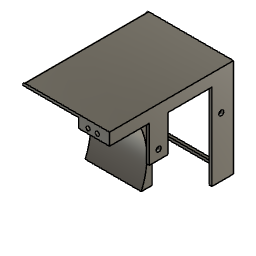
왼쪽 중앙 범퍼 (Autodesk Fusion 360 design; units mm, degrees)
Autodesk Fusion 360 part; units mm, degrees
sketch "스케치1" plane through (0, 0, 0) normal (0, 1, 0) x (1, 0, 0)
  line L0 (-46.5, -52.5) -> (46.5, -52.5)
  line L1 (46.5, -52.5) -> (46.5, 52.5)
  line L2 (46.5, 52.5) -> (-46.5, 52.5)
  line L3 (-46.5, 52.5) -> (-46.5, -52.5)
  line L4 (-46.5, -52.5) -> (46.5, 52.5) construction
  line L5 (46.5, -52.5) -> (-46.5, 52.5) construction
  line L6 (0, -52.5) -> (0, -47.5)
  line L7 (0, 52.5) -> (0, 49.5)
  line L8 (46.5, 0) -> (38.5, 0)
  line L9 (-46.5, 0) -> (-40.5, 0)
  line L10 (-40.5, 0) -> (-40.5, -47.5)
  line L11 (-40.5, -47.5) -> (38.5, -47.5)
  line L12 (38.5, -47.5) -> (38.5, 49.5)
  line L13 (38.5, 49.5) -> (-40.5, 49.5)
  line L14 (-40.5, 49.5) -> (-40.5, 0)
  dimension "d1" = 105
  dimension "d2" = 93
  dimension "d3" = 5
  dimension "d4" = 3
  dimension "d5" = 8
  dimension "d6" = 6
  constraint horizontal L0
  constraint perpendicular L0 L1
  constraint parallel L0 L2
  constraint parallel L1 L3
  constraint coincident L4 origin
  constraint coincident L5 origin
  constraint midpoint L0 L6.start
  constraint perpendicular L0 L6
  constraint midpoint L2 L7.start
  constraint perpendicular L2 L7
  constraint midpoint L1 L8.start
  constraint perpendicular L1 L8
  constraint midpoint L3 L9.start
  constraint perpendicular L3 L9
  constraint perpendicular L9 L10
  constraint perpendicular L6 L11
  constraint perpendicular L2 L12
  constraint perpendicular L12 L13
  constraint perpendicular L9 L14
  measures "d1" distance of L0.end L1.end
  measures "d2" distance of L1.end L2.end
  measures "d3" distance of L6.start L6.end
  measures "d4" distance of L7.start L7.end
  measures "d5" distance of L8.start L8.end
  measures "d6" distance of L9.start L9.end
extrude "돌출1" add sketch "스케치1" along normal blind 132.5 contours L0 L3 L6 L9 L10 L11 | L0 L1 L6 L8 L11 L12 | L2 L3 L7 L9 L13 L14 | L1 L2 L7 L8 L12 L13
sketch "스케치2" plane through (0, 0, 0) normal (0, -1, 0) x (1, 0, 0)
  line L0 (-40.5, -49.5) -> (-40.5, 47.5)
  line L1 (-40.5, 47.5) -> (38.5, 47.5)
  line L2 (38.5, 47.5) -> (38.5, -49.5)
  line L3 (38.5, -49.5) -> (-40.5, -49.5)
  line L4 (-46.5, 52.5) -> (-46.5, -52.5)
  line L5 (-46.5, -52.5) -> (46.5, -52.5)
  line L6 (46.5, -52.5) -> (46.5, 52.5)
  line L7 (46.5, 52.5) -> (-46.5, 52.5)
  line L8 (-46.5, 52.5) -> (-43.5, 52.5)
  line L9 (-43.5, 52.5) -> (-43.5, 49.5)
  line L10 (-43.5, 49.5) -> (-46.5, 49.5)
  line L11 (-46.5, 49.5) -> (-46.5, 52.5)
  line L12 (46.5, -52.5) -> (43.5, -52.5)
  line L13 (-43.5, 49.5) -> (43.5, 49.5)
  line L14 (43.5, 49.5) -> (43.5, -52.5)
  line L15 (43.5, -52.5) -> (-43.5, -52.5)
  line L16 (-43.5, -52.5) -> (-43.5, 49.5)
  dimension "d9" = 3
  dimension "d10" = 3
  dimension "d11" = 3
  constraint horizontal L8
  constraint vertical L9
  constraint horizontal L10
  constraint vertical L11
  constraint coincident L4.start L7.end
  constraint coincident L5.end L6.start
  constraint perpendicular L6 L12
  constraint horizontal L13
  constraint vertical L14
  constraint horizontal L15
  constraint vertical L16
  measures "d9" distance of L4.start L8.end
  measures "d10" distance of L4.start L10.end
  measures "d11" distance of L5.end L12.end
extrude "돌출2" cut sketch "스케치2" against normal blind 129.5 contours L5 L13 L14 L15 L16
sketch "스케치3" plane through (-46.5, 0, 0) normal (-1, 0, 0) x (0, -1, 0)
  line L0 (0, -52.5) -> (0, 52.5)
  line L1 (0, 52.5) -> (-132.5, 52.5)
  line L2 (-132.5, 52.5) -> (-132.5, -52.5)
  line L3 (-132.5, -52.5) -> (0, -52.5)
  line L4 (0, 52.5) -> (0, -23.5)
  circle A0 centre (0, -23.5) radius 73
  circle A1 centre (0, -23.5) radius 75.5
  line L5 (0, 52.5) -> (-42.5, 52.5)
  line L6 (-42.5, 52.5) -> (-42.5, 35.8528)
  line L7 (-42.5, 35.8528) -> (0, 35.8528)
  line L8 (0, 35.8528) -> (0, 52.5)
  line L9 (0, 52.5) -> (-3, 52.5)
  line L10 (-3, 52.5) -> (-3, 49.4383)
  line L11 (-3, 49.4383) -> (0, 49.4383)
  line L12 (0, 49.4383) -> (0, 52.5)
  line L13 (-66.9925, -52.5) -> (-62.9352, -52.5)
  line L14 (-62.9352, -52.5) -> (-62.9352, -49.5)
  line L15 (-62.9352, -49.5) -> (-66.9925, -49.5)
  line L16 (-66.9925, -49.5) -> (-66.9925, -52.5)
  line L17 (0, 52.5) -> (-75.5, 52.5)
  line L18 (-75.5, 52.5) -> (-75.5, -52.5)
  line L19 (-75.5, -52.5) -> (0, -52.5)
  line L20 (0, -52.5) -> (0, 52.5)
  dimension "d14" = 76
  dimension "d15" = 146
  dimension "d16" = 151
  dimension "d45" = 42.5
  dimension "d46" = 3
  dimension "d50" = 3
  dimension "d71" = 75.5
  constraint coincident L0.end L1.start
  constraint perpendicular L1 L4
  constraint coincident L4.end A0.centre
  constraint concentric A0 A1
  constraint horizontal L5
  constraint vertical L6
  constraint horizontal L7
  constraint vertical L8
  constraint coincident A0 L6.end
  constraint horizontal L9
  constraint vertical L10
  constraint horizontal L11
  constraint vertical L12
  constraint coincident A0 L10.end
  constraint horizontal L13
  constraint vertical L14
  constraint horizontal L15
  constraint vertical L16
  constraint coincident A0 L13.start
  constraint coincident L3 L13.start
  constraint horizontal L17
  constraint vertical L18
  constraint horizontal L19
  constraint vertical L20
  measures "d14" distance of L0.end L4.end
  measures "d15" diameter of A0
  measures "d16" diameter of A1
  measures "d45" distance of L0.end L5.end
  measures "d46" distance of L0.end L9.end
  measures "d50" distance of L13.start L15.end
  measures "d71" distance of L0.end L17.end
extrude "돌출3" cut sketch "스케치3" against normal blind 10 contours L0 L3 L4 A0 L7 L14 L15 L16 L19 L20 | L3 L13 L14 L15 L16 L19 | L0 L4 A0 L7 L8 L11 L20 | L0 L4 A0 L8 L11 L12 L20
sketch "스케치4" plane through (0, 132.5, 0) normal (0, 1, 0) x (-1, 0, 0)
  line L0 (40.5, 47.5) -> (40.5, -49.5)
  line L1 (40.5, -49.5) -> (-38.5, -49.5)
  line L2 (-38.5, -49.5) -> (-38.5, 47.5)
  line L3 (-38.5, 47.5) -> (40.5, 47.5)
  line L4 (46.5, -52.5) -> (46.5, 52.5)
  line L5 (46.5, 52.5) -> (-46.5, 52.5)
  line L6 (-46.5, 52.5) -> (-46.5, -52.5)
  line L7 (-46.5, -52.5) -> (46.5, -52.5)
  line L8 (-38.5, -49.5) -> (-38.5, -6.5)
  line L9 (-38.5, -6.5) -> (-28.5, -6.5)
  line L10 (-28.5, -6.5) -> (-28.5, 3.5)
  line L11 (-28.5, 3.5) -> (-38.5, 3.5)
  line L12 (-38.5, 3.5) -> (-38.5, -6.5)
  line L13 (40.5, -6.5) -> (30.5, -6.5)
  line L14 (30.5, -6.5) -> (30.5, 3.5)
  line L15 (30.5, 3.5) -> (40.5, 3.5)
  line L16 (40.5, 3.5) -> (40.5, -6.5)
  circle A0 centre (-33.5, -1.5) radius 2.15
  circle A1 centre (35.5, -1.5) radius 2.15
  dimension "d19" = 43
  dimension "d20" = 10
  dimension "d21" = 10
  dimension "d22" = 10
  dimension "d23" = 10
  dimension "d24" = 4.3
  dimension "d25" = 4.3
  constraint coincident L1.end L2.start
  constraint perpendicular L1 L8
  constraint horizontal L9
  constraint vertical L10
  constraint horizontal L11
  constraint vertical L12
  constraint horizontal L13
  constraint vertical L14
  constraint horizontal L15
  constraint vertical L16
  constraint coincident L0 L13.start
  measures "d19" distance of L1.end L8.end
  measures "d20" distance of L8.end L9.end
  measures "d21" distance of L8.end L11.end
  measures "d22" distance of L13.start L13.end
  measures "d23" distance of L13.start L15.end
  measures "d24" diameter of A0
  measures "d25" diameter of A1
extrude "돌출4" add sketch "스케치4" against normal blind 3 contours L0 L13 L14 L15 L16 | L2 L9 L10 L11 L12
sketch "스케치5" plane through (43.5, 0, 0) normal (-1, 0, 0) x (0, -1, 0)
  line L0 (0, -52.5) -> (0, 49.5)
  line L1 (0, 49.5) -> (-129.5, 49.5)
  line L2 (-129.5, 49.5) -> (-129.5, -52.5)
  line L3 (-129.5, -52.5) -> (0, -52.5)
  line L4 (-129.5, 49.5) -> (-109.5, 49.5)
  line L5 (-109.5, 49.5) -> (-109.5, -52.5)
  line L6 (-109.5, -52.5) -> (-129.5, -52.5)
  line L7 (-129.5, -52.5) -> (-129.5, 49.5)
  line L8 (-109.5, 49.5) -> (-62.5, 49.5)
  line L9 (-62.5, 49.5) -> (-42.5, 49.5)
  line L10 (-42.5, 49.5) -> (-42.5, -52.5)
  line L11 (-42.5, -52.5) -> (-62.5, -52.5)
  line L12 (-62.5, -52.5) -> (-62.5, 49.5)
  line L13 (-42.5, 49.5) -> (-42.5, 20.5)
  line L14 (-109.5, 20.5) -> (-129.5, 20.5)
  line L15 (-129.5, 20.5) -> (-129.5, 0.5)
  line L16 (-129.5, 0.5) -> (-109.5, 0.5)
  line L17 (-109.5, 0.5) -> (-109.5, 20.5)
  circle A0 centre (-119.5, 10.5) radius 2.65
  line L18 (-42.5, 20.5) -> (-62.5, 20.5)
  line L19 (-62.5, 20.5) -> (-62.5, 0.5)
  line L20 (-62.5, 0.5) -> (-42.5, 0.5)
  line L21 (-42.5, 0.5) -> (-42.5, 20.5)
  circle A1 centre (-52.5, 10.5) radius 2.65
  dimension "d28" = 20
  dimension "d29" = 47
  dimension "d30" = 20
  dimension "d31" = 29
  dimension "d33" = 20
  dimension "d34" = 20
  dimension "d36" = 5.3
  dimension "d41" = 20
  dimension "d42" = 5.3
  constraint horizontal L4
  constraint vertical L5
  constraint horizontal L6
  constraint vertical L7
  constraint coincident L1.end L2.start
  constraint perpendicular L5 L8
  constraint horizontal L9
  constraint vertical L10
  constraint horizontal L11
  constraint vertical L12
  constraint perpendicular L1 L13
  constraint horizontal L14
  constraint vertical L15
  constraint horizontal L16
  constraint vertical L17
  constraint coincident L5 L14.start
  constraint horizontal L18
  constraint vertical L19
  constraint horizontal L20
  constraint vertical L21
  measures "d28" distance of L1.end L4.end
  measures "d29" distance of L4.end L8.end
  measures "d30" distance of L8.end L9.end
  measures "d31" distance of L9.end L13.end
  measures "d33" distance of L14.start L14.end
  measures "d34" distance of L14.start L16.end
  measures "d36" diameter of A0
  measures "d41" distance of L13.end L20.end
  measures "d42" diameter of A1
extrude "돌출5" cut sketch "스케치5" against normal blind 3 contours L0 L1 L3 L10 L13 L21 | L3 L10 L11 L12 L20 | L1 L3 L5 L8 L12 L17 L19 | A0 | A1
extrude "돌출19" add sketch "스케치3" against normal blind 60 contours L3 A0 A1 L6 L19 | A0 A1 L6 L10 | L3 A1 L18 L19 | L0 L4 A0 A1 L8 L10 L12 L20 | L1 A1 L5 L6 L10 L17 | L1 A1 L6 L17 L18 | L0 L1 L4 A1 L5 L8 L9 L10 L12 L17 L20
extrude "돌출21" add 1 faces at (-24.5, 75.5, 15.5) along direction (0, 1, 0) blind 3
sketch "스케치12" plane through (0, 0, 49.5) normal (0, 0, -1) x (1, 0, 0)
  line L0 (13.5, -78.5) -> (-43.5, -78.5)
  line L1 (-43.5, -78.5) -> (-43.5, -129.5)
  line L2 (-43.5, -129.5) -> (43.5, -129.5)
  line L3 (43.5, -129.5) -> (43.5, -109.5)
  line L4 (43.5, -109.5) -> (46.5, -109.5)
  line L5 (46.5, -109.5) -> (46.5, -62.5)
  line L6 (46.5, -62.5) -> (43.5, -62.5)
  line L7 (43.5, -62.5) -> (43.5, -42.5)
  line L8 (43.5, -42.5) -> (46.5, -42.5)
  line L9 (46.5, -42.5) -> (46.5, 0)
  line L10 (46.5, 0) -> (13.5, 0)
  line L11 (13.5, 0) -> (13.5, -78.5)
  line L12 (46.5, 0) -> (13.5, 0)
  line L13 (13.5, 0) -> (13.5, -3)
  line L14 (13.5, -3) -> (46.5, -3)
  line L15 (46.5, -3) -> (46.5, 0)
  line L16 (43.5, -129.5) -> (46.5, -129.5)
  line L17 (46.5, -129.5) -> (46.5, 0)
  line L18 (46.5, 0) -> (43.5, 0)
  line L19 (43.5, 0) -> (43.5, -129.5)
  dimension "d103" = 3
  constraint horizontal L12
  constraint vertical L13
  constraint horizontal L14
  constraint vertical L15
  constraint coincident L9.end L10.start
  constraint horizontal L16
  constraint vertical L17
  constraint horizontal L18
  constraint vertical L19
  constraint coincident L2.end L3.start
  measures "d103" distance of L9.end L14.end
extrude "돌출22" add sketch "스케치12" along normal blind 10 contours L10 L11 L12 L13 L14 L19 | L9 L10 L12 L14 L15 L17 L18 L19 | L8 L9 L14 L17 L19 | L4 L5 L6 L17 L19
sketch "스케치13" plane through (0, 0, 0) normal (0, -1, 0) x (1, 0, 0)
  line L0 (46.5, 39.5) -> (46.5, 52.5)
  line L1 (46.5, 52.5) -> (-46.5, 52.5)
  line L2 (-46.5, 52.5) -> (-46.5, 49.5)
  line L3 (-46.5, 49.5) -> (13.5, 49.5)
  line L4 (13.5, 49.5) -> (13.5, 39.5)
  line L5 (13.5, 39.5) -> (46.5, 39.5)
  line L6 (46.5, 52.5) -> (43.5, 52.5)
  line L7 (43.5, 52.5) -> (43.5, 39.5)
  line L8 (43.5, 39.5) -> (46.5, 39.5)
  line L9 (46.5, 39.5) -> (46.5, 52.5)
  line L10 (13.5, 39.5) -> (43.5, 39.5)
  line L11 (43.5, 39.5) -> (43.5, 49.5)
  line L12 (43.5, 49.5) -> (13.5, 49.5)
  line L13 (13.5, 49.5) -> (13.5, 39.5)
  line L14 (13.5, 44.5) -> (23.5, 44.5)
  line L15 (23.5, 44.5) -> (33.5, 44.5)
  circle A0 centre (23.5, 44.5) radius 2.15
  circle A1 centre (33.5, 44.5) radius 2.15
  dimension "d106" = 3
  dimension "d107" = 10
  dimension "d108" = 10
  dimension "d109" = 10
  dimension "d110" = 4.3
  dimension "d111" = 4.3
  constraint horizontal L6
  constraint vertical L7
  constraint horizontal L8
  constraint vertical L9
  constraint coincident L0.end L1.start
  constraint horizontal L10
  constraint vertical L11
  constraint horizontal L12
  constraint vertical L13
  constraint coincident L4.end L5.start
  constraint midpoint L13 L14.start
  constraint perpendicular L13 L14
  constraint perpendicular L13 L15
  constraint coincident L14.end L15.start
  constraint coincident L15.end A1.centre
  measures "d106" distance of L0.end L6.end
  measures "d107" distance of L4.end L3.end
  measures "d108" distance of L14.start L14.end
  measures "d109" distance of L14.end L15.end
  measures "d110" diameter of A0
  measures "d111" diameter of A1
extrude "돌출23" cut sketch "스케치13" against normal blind 3 contours L14 L15 A0 | L14 L15 A0 | A1
fillet "필렛2" radius 2.5 1 edges at (-46.5, 66.25, 52.5)
